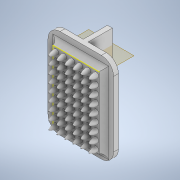
# Autodesk Inventor part: Mold_NewPins_Handle2
Saved by Autodesk Inventor 2021 (Build 250183000, 183)
## iProperties
Created: 2021-04-08
Part Number: Mold_NewPins_Handle2
Material: Generic
Document SubType Name: Modeling
Designer: Olivi
Density: 1 g/cm^3
Appearance: Default
Author: Olivi
Autodesk Inventor part; units mm, degrees
ref_plane "YZ Plane" through (0, 0, 0) normal (1, 0, 0) x (0, 1, 0)
sketch "Sketch1" plane through (0, 0, 0) normal (0, 0, 1) x (1, 0, 0)
  line L0 (0, 0) -> (19.1, 0)
  line L1 (19.1, 0) -> (19.1, 29.4)
  line L2 (19.1, 29.4) -> (0, 29.4)
  line L3 (0, 29.4) -> (0, 0)
  dimension "d0" = 19.1
  dimension "d1" = 29.4
  constraints: 8 end point, 2 horizontal, 2 perpendicular
  measures "d0" distance of L0.start L0.end
  measures "d1" distance of L0.end L1.end
extrude "Extrusion1" add sketch "Sketch1" along normal blind 2
sketch "Sketch2" plane through (0, 0, 2) normal (0, 0, 1) x (1, 0, 0)
  line L0 (0, 29.4) -> (0, 0) projected
  line L1 (19.1, 29.4) -> (0, 29.4) projected
ref_plane "Work Plane1" through (0, 0, 5) normal (0, 0, 1) x (1, 0, 0)
ref_plane "Work Plane2" through (0, 0, 4.5) normal (0, 0, 1) x (1, 0, 0)
sketch "Sketch6" plane through (0, 0, 0) normal (0, 0, -1) x (-1, 0, 0)
  line L0 (0, 29.4) -> (0, 0) projected
  line L1 (0, 15.2241) -> (0, -3.2759)
  line L2 (0, -3.2759) -> (-19.1, -3.2759)
  line L3 (-19.1, 0) -> (-19.1, 29.4) projected
  line L4 (-19.1, -3.2759) -> (-19.1, 33.7241)
  line L5 (-19.1, 33.7241) -> (0, 33.7241)
  line L6 (0, 33.7241) -> (0, -3.2759)
  line L7 (-9.55, -3.2759) -> (3.95, -3.2759)
  line L8 (3.95, -3.2759) -> (3.95, 33.7241)
  line L9 (3.95, 33.7241) -> (-23.05, 33.7241)
  line L10 (-23.05, 33.7241) -> (-23.05, -3.2759)
  line L11 (-23.05, -3.2759) -> (-19.1, -3.2759)
  dimension "d41" = 13.5
  dimension "d42" = 27
  constraints: 20 end point, 4 perpendicular, 3 point on line, 2 collinear, 1 horizontal, 1 midpoint, 1 vertical
  measures "d41" distance of L7.start L7.end
  measures "d42" distance of L8.end L9.end
extrude "Extrusion4" add sketch "Sketch6" along normal blind 2
fillet "Fillet3" radius 5 4 edges at (23.05, -3.2759, -1) (-3.95, -3.2759, -1) (23.05, 33.7241, -1) (-3.95, 33.7241, -1)
sketch "Sketch8" plane through (0, 0, -2) normal (0, 0, -1) x (-1, 0, 0)
  line L0 (3.95, 1.7241) -> (3.95, 28.7241)
  line L1 (-23.05, 28.7241) -> (-23.05, 1.7241) projected
  line L2 (-18.05, -3.2759) -> (-1.05, -3.2759) projected
  line L3 (3.95, 1.7241) -> (3.95, 28.7241) projected
  arc A0 (-18.05, 33.7241) -> (-23.05, 28.7241) centre (-18.05, 28.7241) ccw projected
  line L4 (-1.05, 33.7241) -> (-18.05, 33.7241) projected
  line L5 (-23.05, 28.7241) -> (-23.05, 1.7241) projected
  line L6 (3.95, 1.7241) -> (3.95, 28.7241) projected
  line L7 (3.95, 14) -> (3.95, 16)
  line L8 (-18.05, -3.2759) -> (-1.05, -3.2759) projected
  line L9 (-9.55, -3.2759) -> (-10.55, -3.2759)
  line L10 (-10.55, -3.2759) -> (-10.55, 33.7241)
  line L11 (-10.55, 33.7241) -> (-8.55, 33.7241)
  line L12 (-8.55, 33.7241) -> (-8.55, -3.2759)
  line L13 (-9.55, -3.2759) -> (-8.55, -3.2759)
  point P0 (0, 0)
  point P1 (-21.05, 1.7241)
  dimension "d57" = 1
  dimension "d58" = 2
  constraints: 14 end point, 6 point on line, 3 perpendicular, 1 midpoint
  measures "d57" distance of L9.start L9.end
  measures "d58" distance of L10.end L11.end
extrude "Extrusion5" add sketch "Sketch8" along normal blind 10
fillet "Fillet4" radius 2 4 edges at (19.1, 14.7, 0) (9.55, 29.4, 0) (0, 14.7, 0) (9.55, 0, 0)
ref_plane "Work Plane3" through (1.05, 27.7241, 0) normal (0, 1, 0) x (1, 0, 0)
sketch "Sketch9" plane through (1.05, 27.7241, 0) normal (0, 1, 0) x (1, 0, 0)
  line L0 (-1.05, -2) -> (18.05, -2) projected
  line L1 (-0.5791, -2) -> (0.4009, -2)
  line L2 (-0.5791, -2) -> (0.4009, -2)
  line L3 (0.4009, -2) -> (0.4009, -5)
  line L4 (0.4009, -5) -> (0.2509, -5)
  arc A0 (-0.5791, -2) -> (0.2509, -5) centre (4.807, -2.1247) ccw
  point P0 (-1.05, 0)
  dimension "d60" = 0.98
  dimension "d62" = 3
  dimension "d63" = 0.15
  constraints: 8 end point, 2 horizontal, 2 point on circle, 2 point on line, 1 centre point, 1 perpendicular
  measures "d60" distance of L1.start L1.end
  measures "d62" distance of L1.end L3.end
  measures "d63" distance of L3.end L4.end
revolve "Revolution1" add sketch "Sketch9" angle 360 about axis through (1.4509, 27.7241, 2) along (0, 0, 1)
pattern_linear "Rectangular Pattern2" count 6 spacing 3.3 along (1, 0, 0) count 9 spacing 3.3 along (0, -1, 0) of "Revolution1"
body "Solid1"
